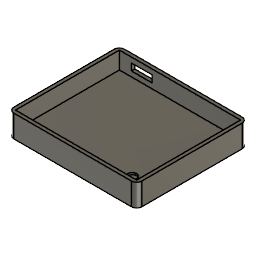
Bottom case (Autodesk Fusion 360 design; units mm, degrees)
part number: 2026-07-07-17-42-05-729
Autodesk Fusion 360 part; units mm, degrees
sketch "Sketch3" plane through (0, 0, 0) normal (0, 0, 1) x (1, 0, 0)
  line L0 (0, 0) -> (74.4, 0)
  line L1 (74.4, 0) -> (74.4, -64.4)
  line L2 (74.4, -64.4) -> (0, -64.4)
  line L3 (0, -64.4) -> (0, 0)
  dimension "d8" = 74.4
  dimension "d9" = 64.4
  constraint horizontal L0
  constraint vertical L1
  constraint horizontal L2
  constraint vertical L3
  constraint coincident L0.start L3.end
  measures "d8" distance of L0.start L0.end
  measures "d9" distance of L0.start L2.end
extrude "Extrude2" add sketch "Sketch3" along normal blind 3
sketch "Sketch4" plane through (0, 0, 3) normal (0, 0, 1) x (-1, 0, 0)
  line L0 (0, 64.4) -> (-74.4, 64.4)
  line L1 (-74.4, 64.4) -> (-74.4, 0)
  line L2 (-74.4, 0) -> (0, 0)
  line L3 (0, 0) -> (0, 64.4)
  line L4 (0, 0) -> (-74.4, 0)
  line L5 (-74.4, 0) -> (-74.4, 2)
  line L6 (-74.4, 2) -> (0, 2)
  line L7 (0, 2) -> (0, 0)
  line L8 (-74.4, 0) -> (-72.4, 0)
  line L9 (-72.4, 0) -> (-72.4, 64.4)
  line L10 (-72.4, 64.4) -> (-74.4, 64.4)
  line L11 (-74.4, 64.4) -> (-74.4, 0)
  line L12 (0, 0) -> (-2, 0)
  line L13 (-2, 0) -> (-2, 64.4)
  line L14 (-2, 64.4) -> (0, 64.4)
  line L15 (0, 64.4) -> (0, 0)
  line L16 (0, 64.4) -> (-74.4, 64.4)
  line L17 (-74.4, 64.4) -> (-74.4, 62.4)
  line L18 (-74.4, 62.4) -> (0, 62.4)
  line L19 (0, 62.4) -> (0, 64.4)
  dimension "d12" = 2
  dimension "d13" = 2
  dimension "d14" = 2
  dimension "d15" = 2
  constraint horizontal L4
  constraint vertical L5
  constraint horizontal L6
  constraint vertical L7
  constraint coincident L2.end L3.start
  constraint horizontal L8
  constraint vertical L9
  constraint horizontal L10
  constraint vertical L11
  constraint coincident L1.end L2.start
  constraint horizontal L12
  constraint vertical L13
  constraint horizontal L14
  constraint vertical L15
  constraint horizontal L16
  constraint vertical L17
  constraint horizontal L18
  constraint vertical L19
  constraint coincident L0.start L3.end
  measures "d12" distance of L2.end L6.end
  measures "d13" distance of L1.end L8.end
  measures "d14" distance of L2.end L12.end
  measures "d15" distance of L0.start L18.end
extrude "Extrude3" add sketch "Sketch4" along normal blind 10 contours L0 L3 L13 L14 L15 L16 L18 L19 | L0 L9 L13 L16 L18 | L3 L6 L13 L15 L18 | L0 L1 L9 L10 L11 L16 L17 L18 | L2 L3 L4 L6 L7 L12 L13 L15 | L1 L6 L9 L11 L18 | L2 L4 L6 L9 L13 | L1 L2 L4 L5 L6 L8 L9 L11
sketch "Sketch6" plane through (0, 0, 0) normal (0, 1, 0) x (-1, 0, 0)
  line L0 (-74.4, 0) -> (0, 0)
  line L1 (0, 0) -> (0, 13)
  line L2 (0, 13) -> (-74.4, 13)
  line L3 (-74.4, 13) -> (-74.4, 0)
  line L4 (-8.3, 5) -> (-22.3, 5)
  line L5 (-22.3, 5) -> (-22.3, 9)
  line L6 (-22.3, 9) -> (-8.3, 9)
  line L7 (-8.3, 9) -> (-8.3, 5)
  dimension "d23" = 14
  dimension "d24" = 8.3
  dimension "d25" = 5
  constraint horizontal L4
  constraint vertical L5
  constraint horizontal L6
  constraint vertical L7
  measures "d23" distance of L4.start L4.end
  measures "d24" distance of L1 L7
  measures "d25" distance of L0 L4
fillet "Fillet1" radius 3 4 edges at (74.4, -64.4, 6.5) (74.4, 0, 6.5) (0, 0, 6.5) (0, -64.4, 6.5)
sketch "Sketch7" plane through (0, 0, 3) normal (0, 0, 1) x (-1, 0, 0)
  line L0 (-2, 62.4) -> (-72.4, 62.4)
  line L1 (-72.4, 62.4) -> (-72.4, 2)
  line L2 (-72.4, 2) -> (-2, 2)
  line L3 (-2, 2) -> (-2, 62.4)
  circle A0 centre (-62.2, 54.7) radius 2.6
  dimension "d30" = 5.2
  dimension "d31" = 10.2
  dimension "d32" = 7.7
  measures "d30" diameter of A0
  measures "d31" distance of L1 A0.centre
  measures "d32" distance of L0 A0.centre
extrude "Extrude5" add sketch "Sketch7" along normal blind 3 contours A0
sketch "Sketch8" plane through (0, 0, 6) normal (0, 0, 1) x (-1, 0, 0)
  circle A0 centre (-62.2, 54.7) radius 2.6
  circle A1 centre (-62.2, 54.7) radius 2.5
  dimension "d35" = 5
  constraint concentric A0 A1
  measures "d35" diameter of A1
extrude "Extrude6" cut sketch "Sketch8" against normal blind 1 contours A1
sketch "Sketch10" plane through (0, -2, 0) normal (0, -1, 0) x (1, 0, 0)
  line L0 (2, 3) -> (72.4, 3)
  line L1 (72.4, 3) -> (72.4, 13)
  line L2 (72.4, 13) -> (2, 13)
  line L3 (2, 13) -> (2, 3)
  line L4 (9, 6) -> (21, 6)
  line L5 (21, 6) -> (21, 10)
  line L6 (21, 10) -> (9, 10)
  line L7 (9, 10) -> (9, 6)
  dimension "d46" = 12
  dimension "d47" = 4
  dimension "d48" = 3
  dimension "d49" = 7
  constraint horizontal L4
  constraint vertical L5
  constraint horizontal L6
  constraint vertical L7
  measures "d46" distance of L4.start L4.end
  measures "d47" distance of L4.start L6.end
  measures "d48" distance of L0 L4
  measures "d49" distance of L3 L7
extrude "Extrude8" cut sketch "Sketch10" against normal blind 3 contours L4 L5 L6 L7
